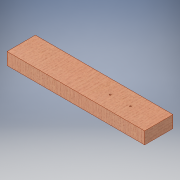
# Autodesk Inventor part: BA02
Saved by Autodesk Inventor 2017 (Build 210142000, 142)
## iProperties
Created: 2018-10-17
Part Number: BA02
Material: Wood (Oak)
Document SubType Name: Modeling
Designer: Administrator
Density: 0.76 g/cm^3
Appearance: White Oak - Natural Medium Gloss
Author: Administrator
Autodesk Inventor part; units mm, degrees
ref_plane "YZ Plane" through (0, 0, 0) normal (1, 0, 0) x (0, 1, 0)
ref_plane "XZ Plane" through (0, 0, 0) normal (0, 1, 0) x (-1, 0, 0)
ref_plane "XY Plane" through (0, 0, 0) normal (0, 0, 1) x (1, 0, 0)
sketch "Sketch1" plane through (0, 0, 0) normal (0, 0, 1) x (1, 0, 0)
  line L0 (0, 0) -> (431.8, 0)
  line L1 (431.8, 0) -> (431.8, 38.1)
  line L2 (431.8, 38.1) -> (0, 38.1)
  line L3 (0, 38.1) -> (0, 0)
  dimension "d0" = 431.8
  dimension "d1" = 38.1
  constraints: 8 end point, 2 parallel, 1 horizontal, 1 perpendicular
  measures "d0" distance of L2.end L1.end
  measures "d1" distance between parallel lines of L0 L2
extrude "Extrusion1" add sketch "Sketch1" along normal blind 88.9
sketch "Sketch4" plane through (0, 38.1, 0) normal (0, 1, 0) x (1, 0, 0)
  circle A0 centre (279.4, -44.45) radius 2.3812
  circle A1 centre (342.9, -44.45) radius 2.3813
  line L0 (279.4, -44.45) -> (342.9, -44.45) construction
  line L1 (431.8, 0) -> (431.8, -88.9) projected
  line L2 (266.7, 0) -> (355.6, 0) construction
  line L3 (355.6, 0) -> (355.6, -88.9) construction
  line L4 (355.6, -88.9) -> (266.7, -88.9) construction
  line L5 (266.7, -88.9) -> (266.7, 0) construction
  line L6 (431.8, 0) -> (0, 0) projected
  line L7 (431.8, -88.9) -> (0, -88.9) projected
  point P0 (311.15, -44.45)
  point P1 (311.15, 0)
  point P2 (266.7, -44.45)
  point P3 (311.15, -88.9)
  dimension "d11" = 4.7625
  dimension "d12" = 4.7625
  dimension "d13" = 63.5
  dimension "d15" = 88.9
  dimension "d16" = 76.2
  constraints: 10 end point, 4 midpoint, 2 centre point, 2 horizontal, 2 parallel, 2 point on line, 1 horizontal alignment, 1 perpendicular, 1 vertical alignment
  measures "d11" diameter of A0
  measures "d12" diameter of A1
  measures "d13" distance of L0.start L0.end
  measures "d15" distance of L2.start L2.end
  measures "d16" distance between parallel lines of L1 L3
extrude "Extrusion3" cut sketch "Sketch4" against normal through all
body "Solid1"
